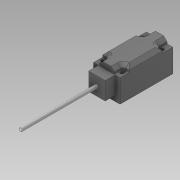
# Autodesk Inventor part: 802K-MSRS11E
Saved by Autodesk Inventor 2020.1 (Build 241239000, 239)
## iProperties
Category: FIRSTChoice
Company: Autodesk Inc.
Created: 2019-12-03
Part Number: 802K-MSRS11E
Material: ABS Plastic
Document SubType Name: Modeling
Designer: Autodesk Inc.
Density: 1.06 g/cm^3
Appearance: Smooth - Black
Catalog Web Link: https://literature.rockwellautomation.com/idc/groups/literature/documents/in/802k-in001_-en-p.pdf
Vendor: Allen Bradley
Author: Autodesk Inc.
Autodesk Inventor part; units mm, degrees
ref_plane "YZ Plane" through (0, 0, 0) normal (1, 0, 0) x (0, 1, 0)
ref_plane "XZ Plane" through (0, 0, 0) normal (0, 1, 0) x (-1, 0, 0)
sketch "Sketch1" plane through (0, 0, 0) normal (0, 0, 1) x (1, 0, 0)
  line L0 (0, 0) -> (80, 0)
  line L1 (80, 0) -> (80, 43)
  line L2 (80, 43) -> (0, 43)
  line L3 (0, 43) -> (0, 0)
  dimension "d0" = 80
  dimension "d1" = 43
  constraints: 8 end point, 2 parallel, 1 horizontal, 1 perpendicular
  measures "d0" distance of L2.end L1.end
  measures "d1" distance of L1.end L0.end
extrude "Extrusion1" add sketch "Sketch1" against normal blind 40
sketch "Sketch2" plane through (0, 43, 0) normal (0, 1, 0) x (1, 0, 0)
  line L0 (80, 0) -> (80, 40) projected
  circle A0 centre (69, 5) radius 2.5
  arc A1 (7.5, 7.5) -> (7.5, 2.5) centre (7.5, 5) ccw
  arc A2 (10.5, 2.5) -> (10.5, 7.5) centre (10.5, 5) ccw
  line L1 (7.5, 7.5) -> (10.5, 7.5)
  line L2 (10.5, 2.5) -> (7.5, 2.5)
  arc A3 (68, 37.5) -> (68, 32.5) centre (68, 35) ccw
  arc A4 (69.5, 32.5505) -> (70, 37.5) centre (70, 35) ccw
  line L3 (68, 37.5) -> (70, 37.5)
  line L4 (68, 32.5) -> (70, 32.5)
  point P0 (0, 0)
  point P1 (69, 35)
  point P2 (9, 5)
  point P3 (9, 35)
  dimension "d4" = 11
  dimension "d5" = 30
  dimension "d6" = 5
  dimension "d7" = 60
  dimension "d16" = 5
  dimension "d17" = 5
  dimension "d18" = 5
  dimension "d19" = 1.5
  dimension "d20" = 1.5
  dimension "d24" = 5
  dimension "d25" = 5
  constraints: 9 point on circle, 8 end point, 5 centre point, 4 horizontal alignment, 3 tangent, 2 horizontal, 2 vertical alignment, 1 coincident, 1 parallel
  measures "d4" distance from line of point (69, 35) L0
  measures "d5" distance of point (69, 5) point (69, 35)
  measures "d6" vertical distance of L0.end point (69, 35)
  measures "d7" distance of point (9, 35) point (69, 35)
  measures "d16" diameter of A0
  measures "d17" diameter of A1
  measures "d18" diameter of A2
  measures "d19" distance of A1.centre point (9, 5)
  measures "d20" distance of A2.centre point (9, 5)
  measures "d24" diameter of A3
  measures "d25" diameter of A4
hole "Hole1" at (69, 43, -5) at (9, 43, -35) direction (0, -1, 0) diameter 5 end through all
extrude "Extrusion2" cut sketch "Sketch2" against normal through all contours L1 A2 L2 A1 | L3 A4 L4 A3
sketch "Sketch3" plane through (0, 43, 0) normal (0, 1, 0) x (1, 0, 0)
  arc A0 (64.25, 35) -> (68, 31.25) centre (68, 35) ccw
  line L0 (64.25, 35) -> (64.25, 40)
  line L1 (68, 31.25) -> (80, 31.25)
  line L2 (64.25, 40) -> (80, 40)
  line L3 (80, 40) -> (80, 31.25)
  line L4 (80, 0) -> (80, 40) projected
  arc A1 (13.75, 5) -> (10, 8.75) centre (10, 5) ccw
  line L5 (10, 8.75) -> (0, 8.75)
  line L6 (13.75, 5) -> (13.75, 0)
  line L7 (0, 0) -> (80, 0) projected
  line L8 (0, 0) -> (0, 40) projected
  line L9 (0, 8.75) -> (0, 0)
  line L10 (0, 0) -> (13.75, 0)
  point P0 (9, 5)
  point P1 (69, 5)
  point P2 (69, 35)
  dimension "d29" = 7.5
  dimension "d34" = 7.5
  dimension "d35" = 1
  constraints: 16 end point, 4 point on circle, 2 centre point, 2 horizontal, 2 vertical, 1 coincident, 1 collinear, 1 horizontal alignment, 1 perpendicular, 1 point on line
  measures "d29" diameter of A0
  measures "d34" diameter of A1
  measures "d35" distance of A1.centre point (9, 5)
extrude "Extrusion3" cut sketch "Sketch3" against normal blind 8
ref_plane "Work Plane1" through (0, 0, -20) normal (0, 0, 1) x (1, 0, 0)
mirror "Mirror2" about plane through (0, 0, -20) normal (0, 0, 1) of "Extrusion3"
chamfer "Chamfer1" distance 5 angle 45 14 edges at (39, 43, 0) (39, 43, -40) (5, 43, -8.75) (12.6517, 43, -7.6517) (13.75, 43, -2.5) (12.6517, 43, -32.3483) (5, 43, -31.25) (13.75, 43, -37.5) (74, 43, -31.25) (65.3483, 43, -32.3483) (64.25, 43, -37.5) (74, 43, -8.75) (65.3483, 43, -7.6517) (64.25, 43, -2.5)
sketch "Sketch4" plane through (0, 0, -40) normal (-1, 0, 0) x (0, 0, 1)
  line L0 (7.5, 35) -> (2.5, 35) projected
  line L1 (7.5, 35) -> (32.5, 35)
  line L2 (32.5, 35) -> (32.5, 8.0021)
  line L3 (32.5, 8.0021) -> (7.5, 8.0021)
  line L4 (7.5, 8.0021) -> (7.5, 35)
  line L5 (7.5, 35) -> (2.5, 35) projected
  point P0 (40, 0)
  constraints: 8 end point, 2 parallel, 1 horizontal, 1 perpendicular
extrude "Extrusion4" add sketch "Sketch4" along normal blind 15
sketch "Sketch5" plane through (-15, 0, -40) normal (-1, 0, 0) x (0, 0, 1)
  line L0 (32.5, 35) -> (7.5, 35) projected
  line L1 (32.5, 8.0021) -> (32.5, 35) projected
  circle A0 centre (20, 21.5011) radius 2.5
  point P0 (40, 0)
  point P1 (20, 35)
  point P2 (32.5, 21.5011)
  dimension "d41" = 5
  constraints: 2 midpoint, 1 centre point, 1 coincident, 1 horizontal alignment, 1 vertical alignment
  measures "d41" diameter of A0
extrude "Extrusion5" add sketch "Sketch5" along normal blind 116
chamfer "Chamfer2" distance 1 angle 45 1 edges at (-131, 21.5011, -22.5)
thread "Thread1" size "M5x0.8" class "6g" standard "ANSI Metric M Profile" full length
body "Solid1"
